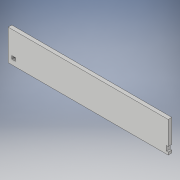
# Autodesk Inventor part: door
Saved by Autodesk Inventor 2017.2 (Build 212233000, 233)
## iProperties
Created: 2017-06-16
Part Number: door
Material: Generic
Document SubType Name: Modeling
Designer: SandeepSH
Density: 1 g/cm^3
Appearance: Default
Author: SandeepSH
Autodesk Inventor part; units mm, degrees
ref_plane "YZ Plane" through (0, 0, 0) normal (1, 0, 0) x (0, 1, 0)
ref_plane "XZ Plane" through (0, 0, 0) normal (0, 1, 0) x (-1, 0, 0)
ref_plane "XY Plane" through (0, 0, 0) normal (0, 0, 1) x (1, 0, 0)
sketch "Sketch1" plane through (0, 0, 0) normal (0, 0, 1) x (1, 0, 0)
  line L0 (0, 0) -> (130, 0)
  line L1 (130, 0) -> (130, 25)
  line L2 (130, 25) -> (0, 25)
  line L3 (0, 25) -> (0, 0)
  line L4 (3, 6.5) -> (6, 6.5)
  line L5 (6, 6.5) -> (6, 4)
  line L6 (6, 4) -> (3, 4)
  line L7 (3, 4) -> (3, 6.5)
  dimension "d0" = 130
  dimension "d1" = 25
  dimension "d2" = 3
  dimension "d3" = 2.5
  dimension "d4" = 3
  dimension "d5" = 4
  constraints: 16 end point, 4 parallel, 2 horizontal, 2 perpendicular
  measures "d0" distance of L2.end L1.end
  measures "d1" distance of L1.end L0.end
  measures "d2" distance of L5.end L6.end
  measures "d3" distance of L4.end L5.end
  measures "d4" distance between parallel lines of L3 L7
  measures "d5" distance between parallel lines of L0 L6
extrude "Extrusion1" add sketch "Sketch1" along normal blind 3
sketch "Sketch2" plane through (0, 0, 3) normal (0, 0, 1) x (1, 0, 0)
  line L0 (130, 0) -> (130, 25) projected
  line L1 (130, 2) -> (128.5, 2)
  line L2 (128.5, 2) -> (128.5, 6)
  line L3 (128.5, 6) -> (130, 6)
  line L4 (130, 6) -> (130, 2)
  line L5 (0, 0) -> (130, 0) projected
  dimension "d8" = 1.5
  dimension "d9" = 4
  dimension "d10" = 2
  constraints: 8 end point, 2 parallel, 1 horizontal, 1 perpendicular, 1 point on line
  measures "d8" distance of L2.end L3.end
  measures "d9" distance of L1.end L2.end
  measures "d10" distance between parallel lines of L5 L1
extrude "Extrusion2" cut sketch "Sketch2" against normal through all
body "Solid1"
